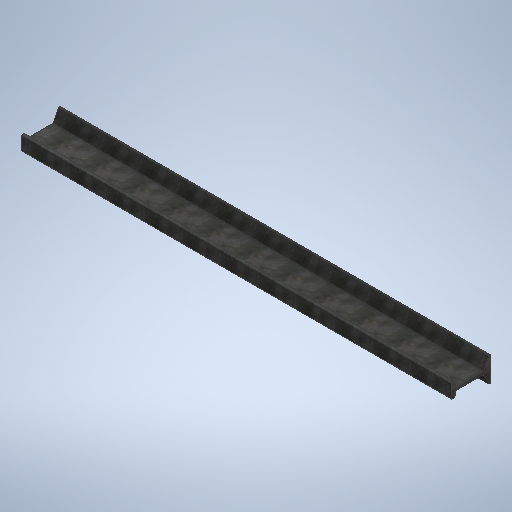
# Autodesk Inventor part: Short I-Beam
Saved by Autodesk Inventor 2025 (Build 290162000, 162)
## iProperties
Created: 2024-06-26
Part Number: Short I-Beam
Material: Steel ASTM A36
Document SubType Name: Modeling
Designer: track
Density: 7.85 g/cm^3
Appearance: Plate
Author: track
Autodesk Inventor part; units mm, degrees
ref_plane "YZ Plane" through (0, 0, 0) normal (1, 0, 0) x (0, 1, 0)
ref_plane "XZ Plane" through (0, 0, 0) normal (0, 1, 0) x (-1, 0, 0)
ref_plane "XY Plane" through (0, 0, 0) normal (0, 0, 1) x (1, 0, 0)
sketch "Sketch1" plane through (0, -4876.8, 165.1) normal (1, 0, 0) x (0, 1, 0)
  line L0 (0, 0) -> (0, -127)
  line L1 (9753.6, 0) -> (9753.6, -127)
  line L2 (9753.6, -152.4) -> (0, -152.4)
  line L3 (5410.2, -152.4) -> (5410.2, -165.1)
  line L4 (5410.2, -165.1) -> (5384.8, -171.45)
  line L5 (5384.8, -171.45) -> (5384.8, -298.45)
  line L6 (5384.8, -298.45) -> (5435.6, -323.85)
  line L7 (5435.6, -323.85) -> (5435.6, -330.2)
  line L8 (5435.6, -330.2) -> (5321.3, -330.2)
  line L9 (5321.3, -330.2) -> (5321.3, -323.85)
  line L10 (5372.1, -298.45) -> (5372.1, -171.45)
  line L11 (5410.2, -152.4) -> (5346.7, -152.4)
  line L12 (5378.45, -325.0091) -> (5378.45, -152.4) construction
  line L13 (5372.1, -171.45) -> (5346.7, -165.1)
  line L14 (5346.7, -165.1) -> (5346.7, -152.4)
  line L15 (5372.1, -298.45) -> (5384.8, -298.45) construction
  line L16 (5321.3, -323.85) -> (5372.1, -298.45)
  point P0 (9753.6, -50.8)
  point P1 (9753.6, -63.5)
  dimension "d8" = 12.7
  dimension "d6" = 6.35
  dimension "d17" = 6.35
  dimension "d12" = 6.35
  dimension "d14" = 50.8
  dimension "d13" = 25.4
  dimension "d16" = 25.4
  dimension "d5" = 25.4
  dimension "d11" = 6.35
  dimension "d10" = 50.8
  dimension "d3" = 90
  dimension "d15" = 127
  dimension "d7" = 177.8
  dimension "d9" = 127
  dimension "d4" = 6.35
  dimension "d2" = 4368.8
  constraints: 32 end point, 5 vertical, 3 parallel, 2 midpoint, 2 point on line, 1 collinear, 3 other
  measures "d8" distance between parallel lines of L10 L5
  measures "d6" distance between parallel lines of L5 L12
  measures "d17" vertical distance of L4.end L3.end
  measures "d12" distance of L6.end L7.end
  measures "d14" horizontal distance of L5.end L6.end
  measures "d13" vertical distance of L5.end L6.end
  measures "d16" horizontal distance of L3.end L4.end
  measures "d5" horizontal distance of L10.end L13.end
  measures "d11" distance of L9.start L9.end
  measures "d10" horizontal distance of L9.end L10.start
  measures "d3" angle of L15 L10
  measures "d15" distance of L4.end L5.end
  measures "d9" distance of L10.start L10.end
  measures "d4" vertical distance of L10.end L13.end
  measures "d2" distance from line of point (9753.6, -63.5) L5
extrude "Extrusion1" add sketch "Sketch1" along normal blind 120.65 and the other way blind 1866.9
body "Solid1"
